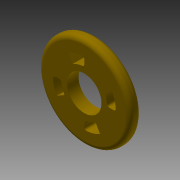
# Autodesk Inventor part: Spool Cap Section Mk1
Saved by Autodesk Inventor 2015 (Build 190159000, 159)
## iProperties
Created: 2016-11-23
Part Number: Spool Cap Section Mk1
Material: Generic
Document SubType Name: Modeling
Designer: Markus
Density: 1 g/cm^3
Appearance: Gold
Author: Markus
Autodesk Inventor part; units mm, degrees
ref_plane "YZ Plane" through (0, 0, 0) normal (1, 0, 0) x (0, 1, 0)
ref_plane "XZ Plane" through (0, 0, 0) normal (0, 1, 0) x (-1, 0, 0)
ref_plane "XY Plane" through (0, 0, 0) normal (0, 0, 1) x (1, 0, 0)
sketch "Sketch1" plane through (0, 0, 0) normal (0, 0, 1) x (1, 0, 0)
  circle A0 centre (0, 0) radius 25.4
  circle A1 centre (0, 0) radius 9.5631
  dimension "d0" = 50.8
  dimension "d4" = 19.1262
  constraints: 2 centre point, 2 coincident
  measures "d0" diameter of A0
  measures "d4" diameter of A1
extrude "Extrusion1" add sketch "Sketch1" along normal blind 6.35
sketch "Sketch2" plane through (0, 0, 6.35) normal (0, 0, 1) x (1, 0, 0)
  circle A0 centre (0, 0) radius 17.5641 construction
  line L0 (0, 17.5641) -> (0, 0) construction
  line L1 (0, 0) -> (-8.782, 15.211) construction
  line L2 (0, 0) -> (0, -17.5641) construction
  line L3 (0, 0) -> (8.7821, -15.211) construction
  circle A1 centre (0, 0) radius 12.7 construction
  arc A2 (0, 12.7) -> (-6.35, 10.9985) centre (0, 0) ccw
  arc A3 (0, 17.5641) -> (-8.782, 15.211) centre (0, 0) ccw
  line L4 (-8.782, 15.211) -> (-6.35, 10.9985)
  line L5 (0, 12.7) -> (0, 17.5641)
  dimension "d5" = 35.1282
  dimension "d6" = 30
  dimension "d7" = 25.4
  constraints: 12 end point, 11 point on circle, 4 centre point, 3 point on line, 3 vertical, 2 coincident, 2 collinear, 2 concentric
  measures "d5" diameter of A0
  measures "d6" angle of L0 L1
  measures "d7" diameter of A1
extrude "Extrusion3" cut sketch "Sketch2" against normal up to surface (6.35 mm away)
pattern_circular "Circular Pattern2" count 4 over 360 about axis through (0, 0, 0) along (0, 0, 1) of "Extrusion3"
fillet "Fillet1" radius 1.27 8 edges at (0, 17.5641, 3.175) (0, 12.7, 3.175) (17.5641, 0, 3.175) (12.7, 0, 3.175) (0, -17.5641, 3.175) (0, -12.7, 3.175) (-17.5641, 0, 3.175) (-12.7, 0, 3.175)
fillet "Fillet2" radius 2.54 2 edges at (-25.4, 0, 0) (-25.4, 0, 6.35)
body "Solid1"
